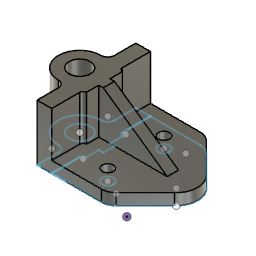
A3 (Autodesk Fusion 360 design; units mm, degrees)
Autodesk Fusion 360 part; units mm, degrees
note: some values were not read from the file. Set by a fixed rule: which sketch regions a step uses.
sketch "bottom" plane through (0, 0, 0) normal (0, 0, 1) x (1, 0, 0)
  line L0 (-22.5627, 0) -> (-67, 0)
  line L1 (-67, 88) -> (-22.5147, 88)
  circle A0 centre (-36, 69) radius 5
  circle A1 centre (-36, 19) radius 5
  line L2 (13.411, 30.589) -> (-13.3703, 3.8076)
  line L3 (13.435, 57.435) -> (-13.3223, 84.1924)
  line L4 (-67, 88) -> (-80, 88)
  line L5 (-80, 0) -> (-67, 0)
  arc A2 (-13.3223, 84.1924) -> (-22.5147, 88) centre (-22.5147, 75) ccw
  arc A3 (12.6084, 29.7863) -> (13.435, 57.435) centre (0, 44) ccw
  arc A4 (-22.5627, 0) -> (-13.3703, 3.8076) centre (-22.5627, 13) ccw
  line L6 (-64, 49) -> (-60, 49)
  line L7 (-60, 49) -> (-60, 39)
  line L8 (-60, 39) -> (-64, 39)
  circle A5 centre (-86, 44) radius 9.5
  line L9 (-64, 60) -> (-64, 49)
  line L10 (-64, 39) -> (-64, 28)
  arc A6 (-86, 63) -> (-85.9962, 25) centre (-86, 44) ccw
  line L11 (-67, 0) -> (-67, 25)
  line L12 (-67, 63) -> (-67, 88)
  line L13 (-67, 0) -> (-67, 25)
  line L14 (-67, 63) -> (-67, 88)
  arc A7 (-64, 28) -> (-67, 25) centre (-64, 25) ccw
  arc A8 (-67, 63) -> (-64, 60) centre (-64, 63) ccw
  line L15 (-85.9962, 25) -> (-86.0038, 25) construction
  arc A9 (-80, 19) -> (-86, 25) centre (-86, 19) ccw
  line L16 (-80, 19) -> (-80, 0)
  line L17 (-80, 88) -> (-80, 69)
  arc A10 (-86, 63) -> (-80, 69) centre (-86, 69) ccw
  dimension "d1" = 67
  dimension "d3" = 19
  dimension "d4" = 19
  dimension "d5" = 10
  dimension "d6" = 10
  dimension "d15" = 45
  dimension "d16" = 13
  dimension "d17" = 13
  dimension "d18" = 13
  dimension "d20" = 3
  dimension "d21" = 38
  dimension "d23" = 4
  dimension "d24" = 10
  dimension "d25" = 39
  dimension "d26" = 6
  dimension "d27" = 6
  dimension "d30" = 19
  dimension "d31" = 38
  dimension "d38" = 6
  dimension "d39" = 6
  constraint horizontal L0
  constraint vertical L11
  constraint horizontal L1
  constraint tangent L2 A4
  constraint tangent L0 A4
  constraint tangent L1 A2
  constraint tangent L3 A2
  constraint horizontal L4
  constraint vertical L17
  constraint horizontal L5
  constraint vertical L13
  constraint coincident L2 A3.start
  constraint vertical L9
  constraint coincident L12.start L13
  constraint horizontal L6
  constraint vertical L7
  constraint horizontal L8
  constraint concentric A5 A6
  constraint collinear L9 L10
  constraint collinear L11 L12
  constraint collinear L13 L14
  constraint collinear L0 L5
  constraint tangent L17 A10
  constraint tangent L15 A9
  constraint coincident A6 A9.end
  constraint coincident A6 L15.end
  measures "d1" distance of origin L0.end
  measures "d3" distance of L1 A0.centre
  measures "d4" distance of L0 A1.centre
  measures "d5" diameter of A0
  measures "d6" diameter of A1
  measures "d15" angle of L0 L2
  measures "d16" radius of A4
  measures "d17" radius of A2
  measures "d18" distance of L1.start L4.end
  measures "d20" distance of L12.start A8.centre
  measures "d21" distance of L12.start L11.end
  measures "d23" distance of L6.start L6.end
  measures "d24" distance of L6.start L8.end
  measures "d25" distance of L1 L6
  measures "d26" diameter of A7
  measures "d27" diameter of A8
  measures "d30" diameter of A5
  measures "d31" diameter of A6
  measures "d38" radius of A10
  measures "d39" radius of A9
extrude "Extrude1" add sketch "bottom" along normal blind 10
extrude "Extrude2" cut sketch "bottom" along normal blind 40 contours L4 L5 L6 L7 L8 L9 L10 A6 L11 L12 L13 L14 A7 A8 A9 L16 L17 A10
extrude "Extrude3" add sketch "bottom" along normal blind 40 contours L4 L5 L6 L7 L8 L9 L10 A6 L11 L12 L13 L14 A7 A8 A9 L16 L17 A10
extrude "Extrude4" add 1 faces at (-71.3333, 73.3333, 40) along direction (0, 0, 1) blind 10
sketch "triangle" plane through (0, 0, 0) normal (0, -1, 0) x (1, 0, 0)
  line L0 (-80, 0) -> (-22.5627, 0)
  line L1 (-22.5627, 0) -> (-22.5627, 10)
  line L2 (-22.5627, 10) -> (-67, 10)
  line L3 (-67, 10) -> (-67, 50)
  line L4 (-67, 50) -> (-80, 50)
  line L5 (-80, 50) -> (-80, 0)
  line L6 (-60, 10) -> (-3, 10)
  line L7 (-60, 10) -> (-60, 50)
  line L8 (-60, 50) -> (-3, 10)
  dimension "d42" = 57
  constraint coincident L2 L6.start
  constraint perpendicular L1 L6
  constraint perpendicular L2 L7
  measures "d42" distance of L6.start L6.end
extrude "Extrude5" add sketch "triangle" along normal blind -49 and the other way blind 39 contours L2 L6 L7 L8
named bodies: "A3 body"
